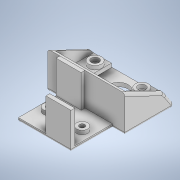
# Autodesk Inventor part: threadedRodMountT
Saved by Autodesk Inventor 2020 (Build 240168000, 168)
## iProperties
Created: 2020-01-08
Part Number: threadedRodMountT
Material: Generic
Document SubType Name: Modeling
Designer: PAB
Density: 1 g/cm^3
Appearance: Default
Author: PAB
Autodesk Inventor part; units mm, degrees
ref_plane "YZ Plane" through (0, 0, 0) normal (1, 0, 0) x (0, 1, 0)
ref_plane "XZ Plane" through (0, 0, 0) normal (0, 1, 0) x (-1, 0, 0)
ref_plane "XY Plane" through (0, 0, 0) normal (0, 0, 1) x (1, 0, 0)
sketch "Sketch1" plane through (0, 0, 0) normal (0, 1, 0) x (-1, 0, 0)
  line L0 (20.5, 16.2) -> (-20.5, 16.2)
  line L1 (-20.5, 16.2) -> (-20.5, -16.2)
  line L2 (-20.5, -16.2) -> (20.5, -16.2)
  line L3 (20.5, -16.2) -> (20.5, 16.2)
  point P0 (0, 0)
  dimension "d0" = 41
  dimension "d1" = 32.4
  constraints: 8 end point, 2 parallel, 1 horizontal, 1 perpendicular
  measures "d0" distance of L2.end L1.end
  measures "d1" distance of L1.end L0.end
extrude "Extrusion1" add sketch "Sketch1" along normal blind 3
sketch "Sketch3" plane through (0, 3, 0) normal (0, 1, 0) x (1, 0, 0)
  line L0 (-20.5, -16.2) -> (20.5, -16.2) projected
  line L1 (-20.5, 16.2) -> (-20.5, -16.2) projected
  line L2 (20.5, -16.2) -> (-20.5, -16.2)
  line L3 (-20.5, -16.2) -> (-20.5, -13.2)
  line L4 (-20.5, -13.2) -> (20.5, -13.2)
  line L5 (20.5, -13.2) -> (20.5, -16.2)
  line L6 (20.5, 16.2) -> (-20.5, 16.2) projected
  line L7 (20.5, 16.2) -> (-20.5, 16.2)
  line L8 (-20.5, 16.2) -> (-20.5, 13.2)
  line L9 (-20.5, 13.2) -> (20.5, 13.2)
  line L10 (20.5, 13.2) -> (20.5, 16.2)
  point P0 (0, 0)
  dimension "d8" = 3
  dimension "d9" = 3
  constraints: 16 end point, 4 parallel, 2 horizontal, 2 perpendicular, 2 point on line
  measures "d8" distance of L2.end L3.end
  measures "d9" distance of L8.end L7.end
extrude "Extrusion3" add sketch "Sketch3" along normal blind 25.4
sketch "Sketch4" plane through (20.5, 0, -16.2) normal (0, 0, -1) x (-1, 0, 0)
  line L0 (41, 3) -> (0, 3) projected
  line L1 (0, 28.4) -> (41, 28.4) projected
  line L2 (0, 3) -> (21.5, 3)
  line L3 (21.5, 3) -> (21.5, 28.4)
  line L4 (21.5, 28.4) -> (0, 28.4)
  line L5 (0, 28.4) -> (0, 3)
  point P0 (20.5, 0)
  dimension "d12" = 21.5
  constraints: 8 end point, 2 parallel, 1 horizontal, 1 perpendicular, 1 point on line
  measures "d12" distance of L4.end L3.end
extrude "Extrusion4" cut sketch "Sketch4" against normal blind 3
sketch "Sketch5" plane through (-20.5, 0, 16.2) normal (0, 0, 1) x (1, 0, 0)
  line L0 (41, 28.4) -> (0, 28.4) projected
  line L1 (19.5, 3) -> (41, 3) projected
  line L2 (0, 28.4) -> (21.5, 28.4)
  line L3 (21.5, 28.4) -> (21.5, 3)
  line L4 (21.5, 3) -> (0, 3)
  line L5 (0, 3) -> (0, 28.4)
  point P0 (20.5, 0)
  dimension "d15" = 21.5
  constraints: 8 end point, 2 parallel, 1 horizontal, 1 perpendicular, 1 point on line
  measures "d15" distance of L3.end L4.end
extrude "Extrusion5" cut sketch "Sketch5" against normal blind 3
sketch "Sketch6" plane through (0, 3, 0) normal (0, 1, 0) x (1, 0, 0)
  circle A0 centre (13, 0) radius 4.25
  circle A1 centre (-13, 0) radius 4.25
  point P0 (0, 0)
  dimension "d20" = 8.5
  dimension "d21" = 8.5
  constraints: 2 centre point
  measures "d20" diameter of A0
  measures "d21" diameter of A1
extrude "Extrusion6" add sketch "Sketch6" along normal blind 3
sketch "Sketch7" plane through (0, 0, 0) normal (0, -1, 0) x (1, 0, 0)
  circle A0 centre (-13, 0) radius 4.25 projected
  circle A1 centre (-13, 0) radius 2
  circle A2 centre (13, 0) radius 4.25 projected
  circle A3 centre (13, 0) radius 2
  point P0 (0, 0)
  dimension "d24" = 4
  dimension "d25" = 4
  constraints: 2 centre point, 2 coincident
  measures "d24" diameter of A1
  measures "d25" diameter of A3
extrude "Extrusion7" cut sketch "Sketch7" against normal blind 6 contours A1 | A3
sketch "Sketch8" plane through (0, 0, 0) normal (0, -1, 0) x (1, 0, 0)
  circle A0 centre (-13, 0) radius 2 projected
  circle A1 centre (-13, 0) radius 3
  circle A2 centre (13, 0) radius 2 projected
  circle A3 centre (13, 0) radius 3
  point P0 (0, 0)
  dimension "d28" = 6
  dimension "d29" = 6
  constraints: 2 centre point, 2 coincident
  measures "d28" diameter of A1
  measures "d29" diameter of A3
extrude "Extrusion8" cut sketch "Sketch8" against normal blind 3 contours A0 | A1 | A2 | A3
sketch "Sketch9" plane through (20.5, 0, -16.2) normal (0, 0, -1) x (-1, 0, 0)
  line L0 (50.5, 0) -> (-9.5, 0)
  line L1 (-9.5, 0) -> (-9.5, 3)
  line L2 (-9.5, 3) -> (50.5, 3)
  line L3 (50.5, 3) -> (50.5, 0)
  point P0 (20.5, 0)
  dimension "d32" = 60
  dimension "d33" = 3
  constraints: 8 end point, 2 parallel, 1 horizontal, 1 perpendicular
  measures "d32" distance of L1.end L2.end
  measures "d33" distance of L0.end L1.end
extrude "Extrusion9" add sketch "Sketch9" along normal blind 40
sketch "Sketch10" plane through (0, 3, 0) normal (0, 1, 0) x (1, 0, 0)
  line L0 (-20.5, 16.2) -> (-30, 16.2) projected
  line L1 (30, 16.2) -> (30, 56.2) projected
  line L2 (-30, 16.2) -> (30, 16.2)
  line L3 (30, 16.2) -> (30, 19.2)
  line L4 (30, 19.2) -> (-30, 19.2)
  line L5 (-30, 19.2) -> (-30, 16.2)
  line L6 (30, 56.2) -> (-30, 56.2) projected
  line L7 (30, 19.2) -> (27, 19.2)
  line L8 (27, 19.2) -> (27, 56.2)
  line L9 (27, 56.2) -> (30, 56.2)
  line L10 (30, 56.2) -> (30, 19.2)
  line L11 (-30, 19.2) -> (-27, 19.2)
  line L12 (-27, 19.2) -> (-27, 56.2)
  line L13 (-27, 56.2) -> (-30, 56.2)
  line L14 (-30, 56.2) -> (-30, 19.2)
  point P0 (0, 0)
  dimension "d36" = 3
  dimension "d37" = 3
  dimension "d38" = 3
  constraints: 24 end point, 6 parallel, 3 horizontal, 3 perpendicular, 3 point on line
  measures "d36" distance of L3.end L2.end
  measures "d37" distance of L8.end L9.end
  measures "d38" distance of L13.end L12.end
extrude "Extrusion10" add sketch "Sketch10" along normal blind 25.4 contours L0 L5 L4 L1 L2 | L14 L6 L12 L4 | L4 L8 L6 L1
sketch "Sketch11" plane through (27, 3, -56.2) normal (-1, 0, 0) x (0, 0, 1)
  line L0 (7.35, 8) -> (22.35, 8)
  line L1 (22.35, 8) -> (22.35, 5)
  line L2 (22.35, 5) -> (7.35, 5)
  line L3 (7.35, 5) -> (7.35, 8)
  point P0 (56.2, -3)
  dimension "d41" = 15
  dimension "d42" = 3
  constraints: 8 end point, 2 parallel, 1 horizontal, 1 perpendicular
  measures "d41" distance of L1.end L2.end
  measures "d42" distance of L0.end L1.end
extrude "Extrusion11" add sketch "Sketch11" along normal blind 14
sketch "Sketch12" plane through (-27, 3, -19.2) normal (1, 0, 0) x (0, 0, -1)
  line L0 (14.65, 8) -> (29.65, 8) projected
  line L1 (29.65, 5) -> (14.65, 5) projected
  line L2 (14.65, 8) -> (29.65, 8)
  line L3 (29.65, 8) -> (29.65, 5)
  line L4 (29.65, 5) -> (14.65, 5)
  line L5 (14.65, 5) -> (14.65, 8)
  point P0 (-19.2, -3)
  constraints: 8 end point, 2 parallel, 1 horizontal, 1 perpendicular
extrude "Extrusion12" add sketch "Sketch12" along normal blind 14
sketch "Sketch13" plane through (0, 0, 0) normal (0, -1, 0) x (1, 0, 0)
  circle A0 centre (0, -41.35) radius 7.5
  circle A1 centre (18.25, -41.35) radius 2
  circle A2 centre (-18.25, -41.35) radius 2
  point P0 (0, 0)
  dimension "d47" = 15
  dimension "d48" = 4
  dimension "d49" = 4
  constraints: 3 centre point
  measures "d47" diameter of A0
  measures "d48" diameter of A1
  measures "d49" diameter of A2
extrude "Extrusion13" cut sketch "Sketch13" against normal blind 14
sketch "Sketch14" plane through (-27, 11, -33.85) normal (0, 1, 0) x (1, 0, 0)
  circle A0 centre (8.75, 7.5) radius 2 projected
  circle A1 centre (8.75, 7.5) radius 3
  circle A2 centre (8.75, 7.5) radius 5
  circle A3 centre (45.25, 7.5) radius 2 projected
  circle A4 centre (45.25, 7.5) radius 3
  circle A5 centre (45.25, 7.5) radius 5
  point P0 (27, -33.85)
  dimension "d52" = 6
  dimension "d53" = 10
  dimension "d54" = 6
  dimension "d55" = 10
  constraints: 4 centre point, 4 coincident
  measures "d52" diameter of A1
  measures "d53" diameter of A2
  measures "d54" diameter of A4
  measures "d55" diameter of A5
extrude "Extrusion14" add sketch "Sketch14" along normal blind 3 contours A2 | A5
sketch "Sketch15" plane through (0, 0, 0) normal (0, -1, 0) x (1, 0, 0)
  point P0 (0, 0)
sketch "Sketch16" plane through (-30, 0, -16.2) normal (-1, 0, 0) x (0, 0, 1)
  line L0 (-20.15, 14) -> (-30.15, 14) projected
  line L1 (0, 28.4) -> (-30.15, 14)
  line L2 (-30.15, 14) -> (-32.65, 11)
  line L3 (0, 0) -> (-40, 0) projected
  line L4 (-32.65, 11) -> (-40, 0)
  line L5 (-40, 0) -> (-40, 28.4)
  line L6 (-40, 3) -> (-3, 3) projected
  line L7 (-40, 28.4) -> (0, 28.4)
  point P0 (16.2, 0)
  constraints: 10 end point, 2 perpendicular
extrude "Extrusion15" cut sketch "Sketch16" against normal blind 60
fillet "Fillet1" radius 2 14 edges at (-30, 0, -36.2) (0, 0, -56.2) (30, 0, -36.2) (25.25, 0, -16.2) (-25.25, 0, -16.2) (-20.5, 0, 0) (0, 0, 16.2) (20.5, 0, 0) (30, 5.5, -52.525) (30, 21.2, -31.275) (-30, 5.5, -52.525) (-30, 21.2, -31.275) (-30, 12.5, -47.6) (30, 12.5, -47.6)
body "Solid1"
